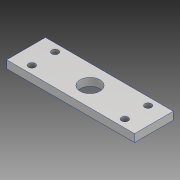
# Autodesk Inventor part: 1222_Former Shaft Plate_V1
Saved by Autodesk Inventor 2020 (Build 240168000, 168)
## iProperties
Created: 2019-09-13
Part Number: 1222_Former Shaft Plate_V1
Material: Aluminum 6061
Document SubType Name: Modeling
Designer: MPI
Density: 2.7 g/cm^3
Appearance: Aluminum - Flat
Author: MPI
Autodesk Inventor part; units mm, degrees
ref_plane "YZ Plane" through (0, 0, 0) normal (1, 0, 0) x (0, 1, 0)
ref_plane "XZ Plane" through (0, 0, 0) normal (0, 1, 0) x (-1, 0, 0)
ref_plane "XY Plane" through (0, 0, 0) normal (0, 0, 1) x (1, 0, 0)
sketch "Sketch1" plane through (0, 0, 0) normal (0, 0, 1) x (1, 0, 0)
  line L0 (-82.5, 25) -> (82.5, 25)
  line L1 (82.5, 25) -> (82.5, -25)
  line L2 (82.5, -25) -> (-82.5, -25)
  line L3 (-82.5, -25) -> (-82.5, 25)
  circle A0 centre (0, 0) radius 12.8
  circle A1 centre (-60, 15) radius 4.25
  circle A2 centre (-60, -15) radius 4.25
  circle A3 centre (60, 15) radius 4.25
  circle A4 centre (60, -15) radius 4.25
  dimension "d0" = 165
  dimension "d1" = 82.5
  dimension "d2" = 25.6
  dimension "d3" = 50
  dimension "d4" = 25
  dimension "d5" = 8.5
  dimension "d6" = 22.5
  dimension "d7" = 22.5
  dimension "d8" = 22.5
  dimension "d9" = 22.5
  dimension "d10" = 10
  dimension "d11" = 10
  dimension "d12" = 10
  dimension "d13" = 10
  constraints: 8 end point, 5 centre point, 3 equal radius, 2 parallel, 1 coincident, 1 horizontal, 1 perpendicular
  measures "d0" distance of L0.start L0.end
  measures "d1" distance from line of point (0, 0) L3
  measures "d2" diameter of A0
  measures "d3" distance of L0.end L1.end
  measures "d4" distance from line of point (0, 0) L0
  measures "d5" diameter of A1
  measures "d6" distance from line of L3 A1.centre
  measures "d7" distance from line of L3 A2.centre
  measures "d8" distance from line of L1 A3.centre
  measures "d9" distance from line of L1 A4.centre
  measures "d10" distance from line of L0 A3.centre
  measures "d11" distance from line of L2 A4.centre
  measures "d12" distance from line of L2 A2.centre
  measures "d13" distance from line of A1.centre L0
extrude "Extrusion1" add sketch "Sketch1" along normal blind 10
body "Solid1"
